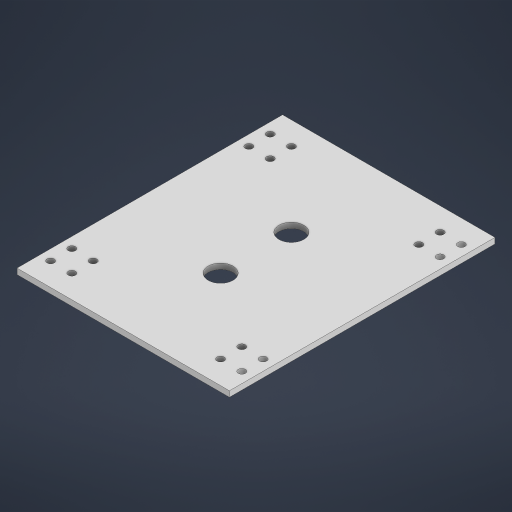
# Autodesk Inventor part: TurretMotorCase_TopPlate
Saved by Autodesk Inventor 2024 (Build 280153000, 153)
## iProperties
Created: 2023-10-26
Part Number: TurretMotorCase_TopPlate
Material: Generic
Document SubType Name: Modeling
Designer: avsar
Density: 1 g/cm^3
Appearance: Default
Author: avsar
Autodesk Inventor part; units mm, degrees
ref_plane "YZ Plane" through (0, 0, 0) normal (1, 0, 0) x (0, 1, 0)
ref_plane "XZ Plane" through (0, 0, 0) normal (0, 1, 0) x (-1, 0, 0)
ref_plane "XY Plane" through (0, 0, 0) normal (0, 0, 1) x (1, 0, 0)
sketch "Sketch1" plane through (0, 0, 0) normal (0, 1, 0) x (-1, 0, 0)
  line L0 (-60, 75) -> (60, 75)
  line L1 (60, 75) -> (60, -75)
  line L2 (60, -75) -> (-60, -75)
  line L3 (-60, -75) -> (-60, 75)
  line L4 (-60, 75) -> (60, -75) construction
  line L5 (60, 75) -> (-60, -75) construction
  point P0 (0, 0)
  dimension "d0" = 120
  dimension "d1" = 150
  constraints: 12 end point, 2 midpoint, 2 parallel, 1 horizontal, 1 perpendicular
  measures "d0" distance of L1.end L2.end
  measures "d1" distance of L0.end L1.end
extrude "Extrusion1" add sketch "Sketch1" along normal blind 3.175
sketch "Sketch2" plane through (0, 3.175, 0) normal (0, 1, 0) x (1, 0, 0)
  circle A0 centre (-48, -56) radius 2.5 construction
  circle A1 centre (-54, -62) radius 2
  circle A2 centre (-42, -62) radius 2
  circle A3 centre (-42, -50) radius 2
  circle A4 centre (-54, -50) radius 2
  line L0 (-60, 75) -> (-60, -75) construction
  line L1 (-60, 0) -> (60, 0) construction
  line L2 (60, -75) -> (60, 75) construction
  line L3 (-60, -75) -> (60, -75) construction
  line L4 (0, -75) -> (0, 72.2302) construction
  circle A5 centre (-54, 62) radius 2
  circle A6 centre (-42, 62) radius 2
  circle A7 centre (-42, 50) radius 2
  circle A8 centre (-54, 50) radius 2
  circle A9 centre (54, -62) radius 2
  circle A10 centre (42, -62) radius 2
  circle A11 centre (42, -50) radius 2
  circle A12 centre (54, -50) radius 2
  circle A13 centre (42, 50) radius 2
  circle A14 centre (54, 50) radius 2
  circle A15 centre (42, 62) radius 2
  circle A16 centre (54, 62) radius 2
  circle A17 centre (0, 0) radius 7 construction
  circle A18 centre (0, 20) radius 7
  circle A19 centre (0, -20) radius 7
  point P0 (0, 0)
  dimension "d4" = 5
  dimension "d5" = 56
  dimension "d6" = 48
  dimension "d7" = 4
  dimension "d8" = 6
  dimension "d9" = 6
  dimension "d12" = 360
  dimension "d14" = 14
  dimension "d17" = 14
  dimension "d20" = 20
  dimension "d21" = 14
  dimension "d22" = 20
  constraints: 20 centre point, 12 symmetric about line, 4 end point, 4 midpoint, 2 vertical alignment, 1 coincident, 1 vertical, 21 other
  measures "d4" diameter of A0
  measures "d5" vertical distance of point (0, 0) A0.centre
  measures "d6" horizontal distance of point (0, 0) A0.centre
  measures "d7" diameter of A1
  measures "d8" horizontal distance of A0.centre A1.centre
  measures "d9" horizontal distance of A0.centre A1.centre
  measures "d14" diameter of A17
  measures "d17" diameter of A18
  measures "d20" distance of point (0, 0) A18.centre
  measures "d21" diameter of A19
  measures "d22" distance of A19.centre point (0, 0)
extrude "Extrusion2" cut sketch "Sketch2" against normal through all
body "Solid1"
